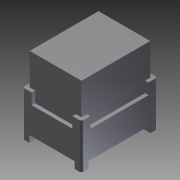
# Autodesk Inventor part: B12APbody
Saved by Autodesk Inventor 2011 SP1 (Build 150282100, 282)
## iProperties
Created: 2013-12-24
Part Number: B12APbody
Catalog Web Link: www.cadenas.de
Description: B Series - Body-
Vendor: NKKSWITCHES
Document SubType Name: Modeling
Designer: PARTuser1
Manufacturer: NKKSWITCHES
Density: 1 g/cm^3
Category: PARTsolutions
Company: NKKSWITCHES
Title: B12APbody
Author: Cadenas PARTsolutions
PSOL_IDENT_0: {$CADENAS_DATA\23d-libs\nkkswitches\toggle\b\parts\b_body.prj},200 {VTYP=3D},{NB=B12APbody},{LINA=B1
PSOL_IDENT_1: 2APbody},{NN=B Series - Body},{DATE=06.03.2009 07:32:50},{GEOMDATE=02.02.2009 06:34:00},{VERSION=},{
PSOL_IDENT_2: LINEID=10},{LINESUBID=-1},{WBVAR=PLS,CRCTS,TGGLS,TRMNLS,CPS,CCLR}  {NB=B12APbody},{LINA=B12APbody},{
PSOL_IDENT_3: KT=DUMMY},{PN=B12AP},{SRS=B},{PLS=1},{CRCTS=2},{CRCTSALG= '2','2 - ON/NONE/ON','3','3 - ON/OFF/ON','
PSOL_IDENT_4: 5','5 - ON/NONE/(ON)','R','R - (ON)/NONE/ON','8','8 - (ON)/OFF/(ON)','9','9 - ON/OFF/(ON)','S','S -
PSOL_IDENT_5: (ON)/OFF/ON' },{TGGLS=A},{TGGLSALG=  'A','A - .394\" (10.0 mm) Bat','J','J - .248\" (6.3 mm) Bat','E
PSOL_IDENT_6: ','E - .394\" (10.0 mm) Flatted','H','H - .248\" (6.3 mm) Flatted','K','K - Snap Top for Paddles' },
PSOL_IDENT_7: {TRMNLS=P},{TRMNLSALG= 'P','P - Straight','B','B - Straight with Bracket', 'H','H - Right Angle with
PSOL_IDENT_8: Bracket','V','V - Vertical with Bracket' ,'W','W - Straight Long' },{CPS=},{CPSALG= '','w/o Cap','-
PSOL_IDENT_9: G','G - .394\" (10.0 mm) Bat Lever Cap' },{CCLR=},{CCLR1= '', 'N/A' }
CNS_NN: B Series - Body
CNS_NB: B12APbody
CNS_NBSYN: $PN.body
CNS_LINA: B12APbody
CNS_PN: B12AP
CNS_SRS: B
CNS_PLS: 1 - SPDT
CNS_CRCTS: 2 - ON/NONE/ON
CNS_CRCTSALG: '2','2 - ON/NONE/ON','3','3 - ON/OFF/ON','5','5 - ON/NONE/(ON)','R','R - (ON)/NONE/ON','8','8 - (ON)/OFF/(ON)','9','9 - ON/OFF/(ON)','S','S - (ON)/OFF/ON'
CNS_TGGLS: A - .394" (10.0 mm) Bat
CNS_TGGLSALG: 'A','A - .394" (10.0 mm) Bat','J','J - .248" (6.3 mm) Bat','E','E - .394" (10.0 mm) Flatted','H','H - .248" (6.3 mm) Flatted','K','K - Snap Top for Paddles'
CNS_TRMNLS: P - Straight
CNS_TRMNLSALG: 'P','P - Straight','B','B - Straight with Bracket', 'H','H - Right Angle with Bracket','V','V - Vertical with Bracket' ,'W','W - Straight Long'
CNS_CPS: w/o Cap
CNS_CPSALG: '','w/o Cap','-G','G - .394" (10.0 mm) Bat Lever Cap'
CNS_CCLR: N/A
CNS_CCLR1: '', 'N/A'
SUPPLIER: NKKSWITCHES
ARTICLENO: B12APbody
BOMINFO: B12APbody
CREATOR: CADENAS GmbH
Autodesk Inventor part; units mm, degrees
sketch "Sketch_1" plane through (0, 0, 0) normal (0, 1, 0) x (-1, 0, 0)
  line L0 (3.4036, -4.1402) -> (3.4036, 4.1402)
  arc A0 (3.4036, 4.1402) -> (3.1496, 4.3942) centre (3.1496, 4.1402) ccw
  line L1 (3.1496, 4.3942) -> (-3.1496, 4.3942)
  arc A1 (-3.1496, 4.3942) -> (-3.4036, 4.1402) centre (-3.1496, 4.1402) ccw
  line L2 (-3.4036, 4.1402) -> (-3.4036, -4.1402)
  arc A2 (-3.4036, -4.1402) -> (-3.1496, -4.3942) centre (-3.1496, -4.1402) ccw
  line L3 (-3.1496, -4.3942) -> (3.1496, -4.3942)
  arc A3 (3.1496, -4.3942) -> (3.4036, -4.1402) centre (3.1496, -4.1402) ccw
  constraints: 8 end point, 8 point on circle, 4 centre point
extrude "Extrusion1" add sketch "Sketch_1" along normal blind 8.8392
sketch "Sketch_2" plane through (0, 8.8392, 0) normal (0, 1, 0) x (1, 0, 0)
  line L0 (-7.3539, 7.1515) -> (-7.3539, -8.5008)
  line L1 (-7.3539, -8.5008) -> (8.5233, -8.5008)
  line L2 (8.5233, -8.5008) -> (8.5233, 7.1515)
  line L3 (8.5233, 7.1515) -> (-7.3539, 7.1515)
  line L4 (-2.9972, -3.9878) -> (2.9972, -3.9878)
  line L5 (2.9972, -3.9878) -> (2.9972, 3.9878)
  line L6 (2.9972, 3.9878) -> (-2.9972, 3.9878)
  line L7 (-2.9972, 3.9878) -> (-2.9972, -3.9878)
  constraints: 16 end point
extrude "Extrusion2" cut sketch "Sketch_2" against normal blind 3.6576
sketch "Sketch_3" plane through (3.4036, 0, 0) normal (1, 0, 0) x (0, 0, -1)
  line L0 (-3.6068, 0) -> (3.6068, 0)
  line L1 (3.6068, 0) -> (3.6068, 0.7874)
  line L2 (3.6068, 0.7874) -> (-3.6068, 0.7874)
  line L3 (-3.6068, 0.7874) -> (-3.6068, 0)
  constraints: 8 end point
extrude "Extrusion3" cut sketch "Sketch_3" against normal blind 6.8072
sketch "Sketch_4" plane through (0, 0, 4.3942) normal (0, 0, 1) x (1, 0, 0)
  line L0 (-2.6162, 0) -> (2.6162, 0)
  line L1 (2.6162, 0) -> (2.6162, 0.7874)
  line L2 (2.6162, 0.7874) -> (-2.6162, 0.7874)
  line L3 (-2.6162, 0.7874) -> (-2.6162, 0)
  constraints: 8 end point
extrude "Extrusion4" cut sketch "Sketch_4" against normal blind 8.7884
sketch "Sketch_5" plane through (3.4036, 0, 0) normal (1, 0, 0) x (0, 0, -1)
  line L0 (-3.3782, 5.1816) -> (-3.3782, 3.9116)
  line L1 (-3.3782, 3.9116) -> (3.3782, 3.9116)
  line L2 (3.3782, 3.9116) -> (3.3782, 5.1816)
  line L3 (3.3782, 5.1816) -> (-3.3782, 5.1816)
  constraints: 8 end point
extrude "Extrusion5" cut sketch "Sketch_5" against normal blind 0.4064
sketch "Sketch_6" plane through (-3.4036, 0, 0) normal (1, 0, 0) x (0, 0, -1)
  line L0 (-3.3782, 5.1816) -> (-3.3782, 3.9116)
  line L1 (-3.3782, 3.9116) -> (3.3782, 3.9116)
  line L2 (3.3782, 3.9116) -> (3.3782, 5.1816)
  line L3 (3.3782, 5.1816) -> (-3.3782, 5.1816)
  constraints: 8 end point
extrude "Extrusion6" cut sketch "Sketch_6" along normal blind 0.4064
sketch "Sketch_7" plane through (0, 0, 4.3942) normal (0, 0, 1) x (1, 0, 0)
  line L0 (-2.3622, 5.1816) -> (-2.3622, 3.9116)
  line L1 (-2.3622, 3.9116) -> (2.3622, 3.9116)
  line L2 (2.3622, 3.9116) -> (2.3622, 5.1816)
  line L3 (2.3622, 5.1816) -> (-2.3622, 5.1816)
  constraints: 8 end point
extrude "Extrusion7" cut sketch "Sketch_7" against normal blind 0.4064
sketch "Sketch_8" plane through (0, 0, -4.3942) normal (0, 0, 1) x (1, 0, 0)
  line L0 (-2.3622, 5.1816) -> (-2.3622, 3.9116)
  line L1 (-2.3622, 3.9116) -> (2.3622, 3.9116)
  line L2 (2.3622, 3.9116) -> (2.3622, 5.1816)
  line L3 (2.3622, 5.1816) -> (-2.3622, 5.1816)
  constraints: 8 end point
extrude "Extrusion8" cut sketch "Sketch_8" along normal blind 0.4064
sketch "Sketch_49" plane through (0, 0.7874, 0) normal (0, 1, 0) x (1, 0, 0)
  line L0 (-2.6162, -3.6068) -> (2.6162, -3.6068)
  line L1 (2.6162, -3.6068) -> (2.6162, 3.6068)
  line L2 (2.6162, 3.6068) -> (-2.6162, 3.6068)
  line L3 (-2.6162, 3.6068) -> (-2.6162, -3.6068)
  constraints: 8 end point
extrude "Extrusion9" cut sketch "Sketch_49" along normal blind 0.0254
ref_plane "black_body_str_XY" through (0, 8.8392, 0) normal (0, -1, 0) x (1, 0, 0)
ref_plane "black_body_str_YZ" through (0, 8.8392, 0) normal (1, 0, 0) x (0, 0, 1)
ref_plane "black_body_str_ZX" through (0, 8.8392, 0) normal (0, 0, 1) x (0, -1, 0)
ref_plane "black_body_ver_rigang_XY" through (0, 0, 9.0678) normal (0, 0, -1) x (1, 0, 0)
ref_plane "black_body_ver_rigang_YZ" through (0, 0, 9.0678) normal (1, 0, 0) x (0, -1, 0)
ref_plane "black_body_ver_rigang_ZX" through (0, 0, 9.0678) normal (0, -1, 0) x (0, 0, -1)
ref_plane "dummy_righ_vert_XY" through (0, 0, 0) normal (0, 0, -1) x (1, 0, 0)
ref_plane "dummy_righ_vert_YZ" through (0, 0, 0) normal (1, 0, 0) x (0, -1, 0)
ref_plane "dummy_righ_vert_ZX" through (0, 0, 0) normal (0, -1, 0) x (0, 0, -1)
ref_plane "dummy_straight_XY" through (0, 0, 0) normal (0, -1, 0) x (1, 0, 0)
ref_plane "dummy_straight_YZ" through (0, 0, 0) normal (1, 0, 0) x (0, 0, 1)
ref_plane "dummy_straight_ZX" through (0, 0, 0) normal (0, 0, 1) x (0, -1, 0)
ref_plane "rigang_vert_trmnls_XY" through (0, 0, 0.8636) normal (0, 0, 1) x (1, 0, 0)
ref_plane "rigang_vert_trmnls_YZ" through (0, 0, 0.8636) normal (1, 0, 0) x (0, 1, 0)
ref_plane "rigang_vert_trmnls_ZX" through (0, 0, 0.8636) normal (0, 1, 0) x (0, 0, 1)
ref_plane "str_trmnls_XY" through (0, 0.8636, 0) normal (0, 1, 0) x (1, 0, 0)
ref_plane "str_trmnls_YZ" through (0, 0.8636, 0) normal (1, 0, 0) x (0, 0, -1)
ref_plane "str_trmnls_ZX" through (0, 0.8636, 0) normal (0, 0, -1) x (0, 1, 0)
body "Solid1"
